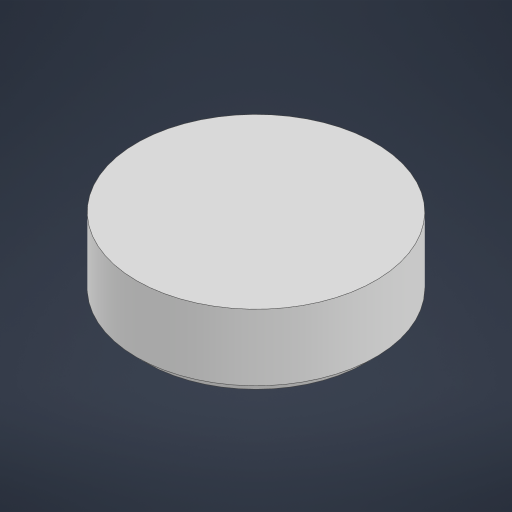
# Autodesk Inventor part: bulkhead
Saved by Autodesk Inventor 2023 (Build 270158000, 158)
## iProperties
Created: 2022-10-07
Part Number: bulkhead
Material: Generic
Document SubType Name: Modeling
Designer: washington
Density: 1 g/cm^3
Appearance: Default
Author: washington
Autodesk Inventor part; units mm, degrees
ref_plane "YZ Plane" through (0, 0, 0) normal (1, 0, 0) x (0, 1, 0)
ref_plane "XZ Plane" through (0, 0, 0) normal (0, 1, 0) x (-1, 0, 0)
ref_plane "XY Plane" through (0, 0, 0) normal (0, 0, 1) x (1, 0, 0)
sketch "Sketch1" plane through (0, 0, 0) normal (1, 0, 0) x (0, 1, 0)
  line L0 (0, 0) -> (15, 0)
  line L1 (15, 0) -> (15, 23.4)
  line L2 (15, 23.4) -> (2, 23.4)
  line L3 (0, 21.4) -> (0, 0)
  line L4 (2, 23.4) -> (0, 21.4)
  point P0 (0, 23.4)
  dimension "d0" = 23.4
  dimension "d1" = 15
  dimension "d2" = 2
  dimension "d3" = 2
  constraints: 10 end point, 2 parallel, 2 point on line, 1 horizontal, 1 perpendicular
  measures "d0" distance of L0.end L1.end
  measures "d1" distance of L1.end point (0, 23.4)
  measures "d2" distance of L2.end point (0, 23.4)
  measures "d3" distance of L3.start point (0, 23.4)
revolve "Revolution1" add sketch "Sketch1" angle 360 about axis through (0, 0, 0) along (0, 1, 0)
equation "\"d3\" = d2"
body "Solid1"
